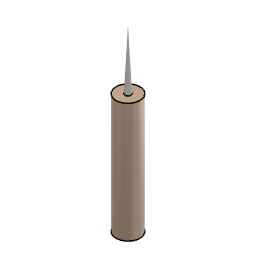
SampleHolder_simple v5 (Autodesk Fusion 360 archive; units mm, degrees)
design "Sample"
Autodesk Fusion 360 part; units mm, degrees
sketch "Skizze1" plane through (0, 0, 0) normal (0, 1, 0) x (1, 0, 0)
  circle A0 centre (0, 0) radius 1
  circle A1 centre (0, 0) radius 0.25
  dimension "d1" = 2
  dimension "d5" = 0.5
  constraint coincident A0.centre A1.centre
  measures "d1" diameter of A0
  measures "d5" diameter of A1
ref_plane "Arbeitsebene1" through (0, 5, 0) normal (0, 1, 0) x (0, 0, 1)
sketch "Skizze2" plane through (0, 5, 0) normal (0, 1, 0) x (1, 0, 0)
extrude "Extrusion1" add sketch "Skizze1" against normal blind 10 contours A0 | A1 makes body 1
loft "Erhebung2" add profiles "Skizze1" section 1 contours A1 section 2 point at (0, 5, 0) separate body makes body 2
